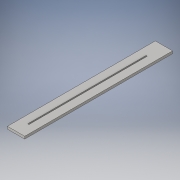
# Autodesk Inventor part: Arm Base
Saved by Autodesk Inventor 2016 (Build 200138000, 138)
## iProperties
Created: 2016-04-23
Part Number: Arm Base
Material: Generic
Document SubType Name: Modeling
Designer: rubenjm
Density: 1 g/cm^3
Appearance: Default
Author: rubenjm
Autodesk Inventor part; units mm, degrees
ref_plane "YZ Plane" through (0, 0, 0) normal (1, 0, 0) x (0, 1, 0)
ref_plane "XZ Plane" through (0, 0, 0) normal (0, 1, 0) x (-1, 0, 0)
ref_plane "XY Plane" through (0, 0, 0) normal (0, 0, 1) x (1, 0, 0)
sketch "Sketch1" plane through (0, 0, 0) normal (0, 1, 0) x (-1, 0, 0)
  line L0 (0, 0) -> (88.9, 0)
  line L1 (88.9, -762) -> (0, -762)
  line L2 (0, -762) -> (0, 0)
  line L3 (88.9, 0) -> (0, 0) construction
  line L4 (0, 0) -> (0, -50.8) construction
  line L5 (88.9, 0) -> (88.9, -762)
  dimension "d0" = 88.9
  dimension "d3" = 50.8
  constraints: 12 end point, 2 horizontal, 2 parallel, 2 perpendicular
  measures "d0" distance of L1.start L1.end
  measures "d3" distance of L4.end L3.end
extrude "Extrusion3" add sketch "Sketch1" along normal blind 12.7
sketch "Sketch2" plane through (0, 12.7, 0) normal (0, 1, 0) x (1, 0, 0)
  line L0 (0, 762) -> (-88.9, 762) construction
  line L1 (-44.45, 762) -> (666.75, 762) construction
  line L2 (-41.275, 63.5) -> (-47.625, 63.5)
  line L3 (-47.625, 63.5) -> (-47.625, 673.1)
  line L4 (-47.625, 673.1) -> (-41.275, 673.1)
  line L5 (-41.275, 673.1) -> (-41.275, 63.5)
  line L6 (-44.45, 63.5) -> (-44.45, 0) construction
  line L7 (-88.9, 0) -> (0, 0) construction
  dimension "d21" = 6.35
  dimension "d22" = 609.6
  dimension "d25" = 63.5
  constraints: 12 end point, 3 midpoint, 2 horizontal, 2 parallel, 1 perpendicular
  measures "d21" distance of L3.end L4.end
  measures "d22" distance of L2.end L3.end
  measures "d25" distance of L6.start L6.end
extrude "Extrusion4" cut sketch "Sketch2" against normal through all
body "Solid3"
